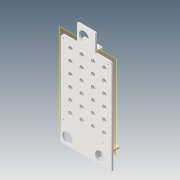
# Autodesk Inventor part: Omniscope_lensmount_v0
Saved by Autodesk Inventor 2022 (Build 260153000, 153)
## iProperties
Created: 2022-05-27
Part Number: Omniscope_lensmount_v0
Material: Generisch
Document SubType Name: Modeling
Designer: diederichbenedict
Density: 1 g/cm^3
Appearance: Vorgabe
Author: diederichbenedict
Autodesk Inventor part; units mm, degrees
ref_plane "YZ Plane" through (0, 0, 0) normal (1, 0, 0) x (0, 1, 0)
ref_plane "XZ Plane" through (0, 0, 0) normal (0, 1, 0) x (-1, 0, 0)
ref_plane "XY Plane" through (0, 0, 0) normal (0, 0, 1) x (1, 0, 0)
ref_plane "Arbeitsebene1" through (0, 0, 0) normal (0, 0, 1) x (1, 0, 0)
sketch "Skizze1" plane through (0, 0, 0) normal (0, 0, 1) x (1, 0, 0)
  arc A0 (-36.75, 55.75) -> (-34.75, 57.75) centre (-36.75, 57.75) ccw projected
  line L0 (-34.75, 57.75) -> (-34.75, 60.25) projected
  arc A1 (-32.75, 62.25) -> (-34.75, 60.25) centre (-32.75, 60.25) ccw projected
  line L1 (-32.75, 62.25) -> (32.25, 62.25) projected
  arc A2 (34.25, 60.25) -> (32.25, 62.25) centre (32.25, 60.25) ccw projected
  line L2 (34.25, 60.25) -> (34.25, 57.25) projected
  arc A3 (34.25, 57.25) -> (36.25, 55.25) centre (36.25, 57.25) ccw projected
  line L3 (36.25, 55.25) -> (39.25, 55.25) projected
  arc A4 (41.25, 53.25) -> (39.25, 55.25) centre (39.25, 53.25) ccw projected
  line L4 (41.25, 53.25) -> (41.25, -58.75) projected
  arc A5 (37.75, -62.25) -> (41.25, -58.75) centre (37.75, -58.75) ccw projected
  line L5 (37.75, -62.25) -> (33.25, -62.25) projected
  arc A6 (31.25, -60.25) -> (33.25, -62.25) centre (33.25, -60.25) ccw projected
  line L6 (31.25, -60.25) -> (31.25, -57.25) projected
  arc A7 (31.25, -57.25) -> (29.25, -55.25) centre (29.25, -57.25) ccw projected
  line L7 (29.25, -55.25) -> (26.25, -55.25) projected
  arc A8 (26.25, -55.25) -> (24.25, -57.25) centre (26.25, -57.25) ccw projected
  line L8 (24.25, -57.25) -> (24.25, -60.25) projected
  arc A9 (22.25, -62.25) -> (24.25, -60.25) centre (22.25, -60.25) ccw projected
  line L9 (22.25, -62.25) -> (-30.5541, -62.25) projected
  arc A10 (-32.5541, -60.25) -> (-30.5541, -62.25) centre (-30.5541, -60.25) ccw projected
  line L10 (-32.5541, -60.25) -> (-32.5541, -56.8048) projected
  arc A11 (-32.5541, -56.8048) -> (-34.5541, -54.8048) centre (-34.5541, -56.8048) ccw projected
  line L11 (-34.5541, -54.8048) -> (-39.25, -54.8048) projected
  arc A12 (-41.25, -52.8048) -> (-39.25, -54.8048) centre (-39.25, -52.8048) ccw projected
  line L12 (-41.25, -52.8048) -> (-41.25, 53.75) projected
  arc A13 (-39.25, 55.75) -> (-41.25, 53.75) centre (-39.25, 53.75) ccw projected
  line L13 (-39.25, 55.75) -> (-36.75, 55.75) projected
  line L14 (42.75, -58.75) -> (42.75, 58.75) projected
  arc A14 (42.75, 58.75) -> (37.75, 63.75) centre (37.75, 58.75) ccw projected
  line L15 (37.75, 63.75) -> (-37.75, 63.75) projected
  arc A15 (-37.75, 63.75) -> (-42.75, 58.75) centre (-37.75, 58.75) ccw projected
  line L16 (-42.75, 58.75) -> (-42.75, -58.75) projected
  arc A16 (-42.75, -58.75) -> (-37.75, -63.75) centre (-37.75, -58.75) ccw projected
  line L17 (-37.75, -63.75) -> (37.75, -63.75) projected
  arc A17 (37.75, -63.75) -> (42.75, -58.75) centre (37.75, -58.75) ccw projected
  circle A18 centre (-37.75, 58.75) radius 1.4 projected
  circle A19 centre (-37.75, -58.75) radius 1.4 projected
  circle A20 centre (37.75, 58.75) radius 1.4 projected
  circle A21 centre (28.25, -59.25) radius 1.4 projected
  point P0 (0, 0)
extrude "Extrusion1" add sketch "Skizze1" along normal blind 3 contours A0 L0 A1 L1 A2 L2 A3 L3 A4 L4 A5 L5 A6 L6 A7 L7 A8 L8 A9 L9 A10 L10 A11 L11 A12 L12 A13 L13 | A17 L17 A16 L16 A15 L15 A14 L14
sketch "Skizze2" plane through (0, 0, 3) normal (0, 0, 1) x (1, 0, 0)
  circle A0 centre (-26.4114, 50.1197) radius 3.8655 construction
  circle A1 centre (-26.4114, 50.1197) radius 3.5
  point P0 (0, 0)
  dimension "d2" = 7
  constraints: 1 centre point, 1 coincident
  measures "d2" diameter of A1
extrude "Extrusion2" cut sketch "Skizze2" against normal through all
pattern_linear "Rechteckige Anordnung1" count 6 spacing 18.9 along (0, -1, 0) count 4 spacing 18.9 along (1, 0, 0) of "Extrusion2"
sketch "Skizze3" plane through (0, 0, 3) normal (0, 0, 1) x (1, 0, 0)
  circle A0 centre (-28.25, -81.65) radius 8.5 projected
  line L0 (-9.25, -66.75) -> (-39.75, -66.75) projected
  line L1 (-39.75, -66.75) -> (-39.75, -93.15) projected
  line L2 (-39.75, -93.15) -> (-9.25, -93.15) projected
  line L3 (-9.25, -93.15) -> (-9.25, -66.75) projected
  circle A1 centre (-3.75, 78.25) radius 8.5 projected
  line L4 (15.25, 93.15) -> (-15.25, 93.15) projected
  line L5 (-15.25, 93.15) -> (-15.25, 66.75) projected
  line L6 (-15.25, 66.75) -> (15.25, 66.75) projected
  line L7 (15.25, 66.75) -> (15.25, 93.15) projected
  circle A2 centre (20.75, -81.65) radius 8.5 projected
  line L8 (39.75, -66.75) -> (9.25, -66.75) projected
  line L9 (9.25, -66.75) -> (9.25, -93.15) projected
  line L10 (9.25, -93.15) -> (39.75, -93.15) projected
  line L11 (39.75, -93.15) -> (39.75, -66.75) projected
  line L12 (-42.75, 58.75) -> (-42.75, -58.75) projected
  line L13 (-42.75, -66.75) -> (-42.75, -58.75)
  line L14 (-42.75, -58.75) -> (-41.9493, -58.75)
  line L15 (-9.25, -93.15) -> (9.25, -93.15)
  arc A3 (37.75, -63.75) -> (42.75, -58.75) centre (37.75, -58.75) ccw projected
  line L16 (42.75, -66.75) -> (42.75, -58.75)
  line L17 (37.75, 63.75) -> (-37.75, 63.75) projected
  line L18 (-15.25, 93.15) -> (15.25, 93.15)
  line L19 (15.25, 93.15) -> (15.25, 63.75)
  line L20 (15.25, 63.75) -> (-15.25, 63.75)
  line L21 (-15.25, 63.75) -> (-15.25, 93.15)
  arc A4 (-42.75, -58.75) -> (-37.75, -63.75) centre (-37.75, -58.75) ccw projected
  circle A5 centre (30.2886, -44.3803) radius 3.5 projected
  circle A6 centre (30.2886, -25.4803) radius 3.5 projected
  circle A7 centre (30.2886, -6.5803) radius 3.5 projected
  circle A8 centre (30.2886, 12.3197) radius 3.5 projected
  circle A9 centre (30.2886, 31.2197) radius 3.5 projected
  circle A10 centre (30.2886, 50.1197) radius 3.5 projected
  circle A11 centre (11.3886, -44.3803) radius 3.5 projected
  circle A12 centre (11.3886, -25.4803) radius 3.5 projected
  circle A13 centre (11.3886, -6.5803) radius 3.5 projected
  circle A14 centre (11.3886, 12.3197) radius 3.5 projected
  circle A15 centre (11.3886, 31.2197) radius 3.5 projected
  circle A16 centre (11.3886, 50.1197) radius 3.5 projected
  circle A17 centre (-7.5114, -44.3803) radius 3.5 projected
  circle A18 centre (-7.5114, -25.4803) radius 3.5 projected
  circle A19 centre (-7.5114, -6.5803) radius 3.5 projected
  circle A20 centre (-7.5114, 12.3197) radius 3.5 projected
  circle A21 centre (-7.5114, 31.2197) radius 3.5 projected
  circle A22 centre (-7.5114, 50.1197) radius 3.5 projected
  circle A23 centre (-26.4114, -44.3803) radius 3.5 projected
  circle A24 centre (-26.4114, -25.4803) radius 3.5 projected
  circle A25 centre (-26.4114, -6.5803) radius 3.5 projected
  circle A26 centre (-26.4114, 12.3197) radius 3.5 projected
  circle A27 centre (-26.4114, 31.2197) radius 3.5 projected
  circle A28 centre (-26.4114, 50.1197) radius 3.5 projected
  arc A29 (42.75, 58.75) -> (37.75, 63.75) centre (37.75, 58.75) ccw projected
  line L22 (37.75, 63.75) -> (-37.75, 63.75) projected
  arc A30 (-37.75, 63.75) -> (-42.75, 58.75) centre (-37.75, 58.75) ccw projected
  line L23 (-42.75, 58.75) -> (-42.75, -58.75) projected
  arc A31 (-42.75, -58.75) -> (-37.75, -63.75) centre (-37.75, -58.75) ccw projected
  line L24 (-37.75, -63.75) -> (37.75, -63.75) projected
  arc A32 (37.75, -63.75) -> (42.75, -58.75) centre (37.75, -58.75) ccw projected
  line L25 (42.75, -58.75) -> (42.75, 58.75) projected
  circle A33 centre (28.25, -59.25) radius 1.4 projected
  circle A34 centre (37.75, 58.75) radius 1.4 projected
  circle A35 centre (-37.75, -58.75) radius 1.4 projected
  circle A36 centre (-37.75, 58.75) radius 1.4 projected
  line L26 (15.25, 93.15) -> (18.25, 93.15)
  line L27 (18.25, 93.15) -> (18.25, 63.75)
  line L28 (18.25, 63.75) -> (15.25, 63.75)
  line L29 (15.25, 63.75) -> (15.25, 93.15)
  line L30 (-15.25, 93.15) -> (-18.25, 93.15)
  line L31 (-18.25, 93.15) -> (-18.25, 63.75)
  line L32 (-18.25, 63.75) -> (-15.25, 63.75)
  line L33 (-15.25, 63.75) -> (-15.25, 93.15)
  line L34 (-39.75, -93.15) -> (-42.75, -93.15)
  line L35 (-42.75, -93.15) -> (-42.75, -58.75)
  line L36 (-42.75, -58.75) -> (-39.75, -58.75)
  line L37 (-39.75, -58.75) -> (-39.75, -93.15)
  line L38 (39.75, -93.15) -> (42.75, -93.15)
  line L39 (42.75, -93.15) -> (42.75, -58.75)
  line L40 (42.75, -58.75) -> (39.75, -58.75)
  line L41 (39.75, -58.75) -> (39.75, -93.15)
  point P0 (0, 0)
  point P1 (15.25, 66.75)
  point P2 (-15.25, 63.75)
  point P3 (41.5171, -62.0377)
  point P4 (42.75, -58.75)
  point P5 (42.75, -58.75)
  point P6 (-41.5171, -62.0377)
  point P7 (42.75, -58.75)
  point P8 (41.5171, -62.0377)
  point P9 (42.75, -58.75)
  dimension "d17" = 3
  dimension "d18" = 3
  constraints: 44 end point, 10 parallel, 6 horizontal, 6 perpendicular, 3 point on line, 1 vertical, 7 other
  measures "d17" distance of L27.end L28.end
  measures "d18" distance of L32.end L31.end
ref_plane "Arbeitsebene2" through (-15.25, 66.75, 0) normal (0, 0, 1) x (1, 0, 0)
extrude "Extrusion3" add sketch "Skizze3" against normal up to surface (3 mm away) contours L3 L2 L1 L0 | L0 L37 A4 L24 A3 L41 L8 L9 L15 L3 | L1 L34 L35 L13 A4 L37 | L37 L36 L14 L12 A30 L17 A29 L25 L40 L41 A3 L24 A4 | A4 L14 L36 L37 | L9 L8 L11 L10 | L11 L41 A3 L16 L39 L38 | L41 L40 A3 | L31 L30 L5 L21 L17 | L21 L6 L19 L17 | L19 L7 L26 L27 L17 | L5 L4 L7 L6 | A5 | A6 | A7 | A8 | A9 | A10 | A11 | A12 | A13 | A14 | A15 | A16 | A17 | A18 | A19 | A20 | A21 | A22 | A23 | A24 | A25 | A26 | A27 | A28 | A33 | A34 | A35 | A36
sketch "Skizze4" plane through (0, 0, 0) normal (0, 0, -1) x (-1, 0, 0)
  circle A0 centre (19.25, -88.65) radius 0.65 projected
  line L0 (9.25, -93.15) -> (9.25, -66.75) projected
  line L1 (9.25, -66.75) -> (39.75, -66.75) projected
  line L2 (-9.25, -66.75) -> (-9.25, -93.15) projected
  line L3 (-39.75, -66.75) -> (-9.25, -66.75) projected
  line L4 (15.25, 66.75) -> (-15.25, 66.75) projected
  line L5 (-37.75, 63.75) -> (37.75, 63.75) projected
  line L6 (-15.25, 66.75) -> (15.25, 66.75)
  line L7 (15.25, 66.75) -> (15.25, 63.75)
  line L8 (15.25, 63.75) -> (-15.25, 63.75)
  line L9 (-15.25, 63.75) -> (-15.25, 66.75)
  line L10 (9.25, -93.15) -> (6.25, -93.15)
  line L11 (6.25, -93.15) -> (6.25, -63.7252)
  line L12 (6.25, -63.7252) -> (9.25, -63.7252)
  line L13 (9.25, -63.7252) -> (9.25, -93.15)
  line L14 (-9.25, -93.15) -> (-6.25, -93.15)
  line L15 (-6.25, -93.15) -> (-6.25, -63.7252)
  line L16 (-6.25, -63.7252) -> (-9.25, -63.7252)
  line L17 (-9.25, -63.7252) -> (-9.25, -93.15)
  line L18 (42.75, 58.75) -> (42.75, -93.15) projected
  line L19 (-42.75, 58.75) -> (-42.75, -93.15) projected
  line L20 (-9.25, -66.75) -> (-39.75, -66.75)
  line L21 (-39.75, -66.75) -> (-39.75, -63.7252)
  line L22 (-39.75, -63.7252) -> (-9.25, -63.7252)
  line L23 (-9.25, -63.7252) -> (-9.25, -66.75)
  line L24 (42.75, 58.75) -> (42.75, -93.15) projected
  line L25 (9.25, -66.75) -> (42.75, -66.75)
  line L26 (42.75, -66.75) -> (42.75, -63.7252)
  line L27 (42.75, -63.7252) -> (9.25, -63.7252)
  line L28 (9.25, -63.7252) -> (9.25, -66.75)
  line L29 (-18.25, 93.15) -> (-18.25, 63.75) projected
  line L30 (18.25, 63.75) -> (18.25, 93.15) projected
  line L31 (-18.25, 93.15) -> (-15.25, 93.15)
  line L32 (-15.25, 93.15) -> (-15.25, 63.75)
  line L33 (-15.25, 63.75) -> (-18.25, 63.75)
  line L34 (-18.25, 63.75) -> (-18.25, 93.15)
  line L35 (18.25, 63.75) -> (37.75, 63.75) projected
  line L36 (18.25, 63.75) -> (15.25, 63.75)
  line L37 (15.25, 63.75) -> (15.25, 93.15)
  line L38 (15.25, 93.15) -> (18.25, 93.15)
  line L39 (18.25, 93.15) -> (18.25, 63.75)
  line L40 (-42.75, -93.15) -> (-42.75, 58.75) projected
  line L41 (-42.75, -93.15) -> (-39.75, -93.15)
  line L42 (-39.75, -93.15) -> (-39.75, -63.7252)
  line L43 (-39.75, -63.7252) -> (-42.75, -63.7252)
  line L44 (-42.75, -63.7252) -> (-42.75, -93.15)
  line L45 (42.75, -93.15) -> (39.75, -93.15)
  line L46 (39.75, -93.15) -> (39.75, -66.75)
  line L47 (39.75, -66.75) -> (42.75, -66.75)
  line L48 (42.75, -66.75) -> (42.75, -93.15)
  point P0 (0, 0)
  point P1 (9.25, -63.7252)
  point P2 (9.25, -66.75)
  point P3 (-9.25, -63.7252)
  point P4 (-42.75, -63.7252)
  point P5 (-9.25, -66.75)
  point P6 (-9.25, -63.7252)
  point P7 (-42.75, -58.75)
  point P8 (42.75, -58.75)
  dimension "d13" = 3
  dimension "d14" = 3
  constraints: 72 end point, 18 parallel, 9 horizontal, 9 perpendicular, 3 point on line, 4 other
  measures "d13" distance of L11.end L12.end
  measures "d14" distance of L16.end L15.end
extrude "Extrusion4" add sketch "Skizze4" along normal blind 10 contours L10 L11 L12 L13 L0 | L13 L27 L18 L25 L1 | L25 L18 L45 L46 | L17 L16 L15 L14 L2 | L3 L21 L22 L17 | L42 L41 L19 L43 L21 | L7 L5 L9 L4 | L37 L38 L30 L5 L7 | L9 L5 L29 L31 L32
